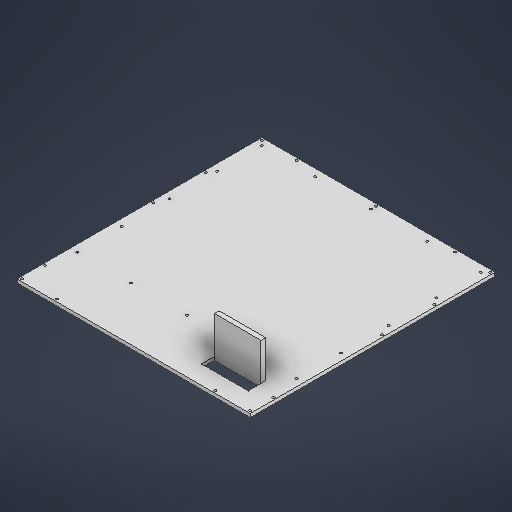
# Autodesk Inventor part: DesignAtasRobot
Saved by Autodesk Inventor 2026.1 (Build 301233020, 233B)
## iProperties
Created: 2025-11-08
Part Number: DesignAtasRobot
Material: Generic
Document SubType Name: Modeling
Designer: FrianVex
Density: 1 g/cm^3
Appearance: Default
Author: FrianVex
Autodesk Inventor part; units mm, degrees
ref_plane "YZ Plane" through (0, 0, 0) normal (1, 0, 0) x (0, 1, 0)
ref_plane "XZ Plane" through (0, 0, 0) normal (0, 1, 0) x (-1, 0, 0)
ref_plane "XY Plane" through (0, 0, 0) normal (0, 0, 1) x (1, 0, 0)
sketch "Sketch1" plane through (0, 0, 0) normal (0, 1, 0) x (-1, 0, 0)
  line L0 (100, -105) -> (-100, -105)
  line L1 (-100, -105) -> (-100, 105)
  line L2 (-100, 105) -> (100, 105)
  line L3 (100, 105) -> (100, -105)
  line L4 (100, -105) -> (-100, 105) construction
  line L5 (-100, -105) -> (100, 105) construction
  line L6 (-42.3092, 89.0348) -> (-82.3092, 89.0348)
  line L7 (-82.3092, 89.0348) -> (-82.3092, 74.0348)
  line L8 (-82.3092, 74.0348) -> (-42.3092, 74.0348)
  line L9 (-42.3092, 74.0348) -> (-42.3092, 89.0348)
  line L10 (-42.3092, 89.0348) -> (-82.3092, 74.0348) construction
  line L11 (-82.3092, 89.0348) -> (-42.3092, 74.0348) construction
  circle A0 centre (98, 83) radius 1
  circle A1 centre (98, 102.9) radius 1
  circle A2 centre (68, 102.9) radius 1
  circle A3 centre (-98, 102.9) radius 1
  circle A4 centre (-68, 102.9) radius 1
  circle A5 centre (98, -10) radius 1
  circle A6 centre (98, -55) radius 1
  circle A7 centre (-98, 83) radius 1
  circle A8 centre (-98, -10) radius 1
  circle A9 centre (-98, -55) radius 1
  circle A10 centre (-98, -102.9) radius 1.0002
  circle A11 centre (98, -102.9) radius 1
  circle A12 centre (-68, -102.9) radius 1
  circle A13 centre (0, -102.9) radius 1
  circle A14 centre (68, -102.9) radius 1
  line L12 (96, 61.2) -> (96, -100.8)
  circle A15 centre (94, -98.8) radius 1
  circle A16 centre (-94, -98.8) radius 1
  circle A17 centre (-94, 59.2) radius 1
  circle A18 centre (94, 59.2) radius 1
  circle A19 centre (94, -60.8) radius 1
  circle A20 centre (94, -19.8) radius 1
  circle A21 centre (94, 21.2) radius 1
  circle A22 centre (-94, -60.8) radius 1
  circle A23 centre (-94, -19.8) radius 1
  circle A24 centre (-94, 21.2) radius 1
  circle A25 centre (0, 59.2) radius 1
  circle A26 centre (0, -98.8) radius 1
  circle A27 centre (-48, 59.2) radius 1
  circle A28 centre (-48, -98.8) radius 1
  circle A29 centre (48, 59.2) radius 1
  circle A30 centre (48, -98.8) radius 1
  point P0 (0, 0)
  point P1 (-62.3092, 81.5348)
  dimension "d0" = 200
  dimension "d1" = 210
  dimension "d2" = 40
  dimension "d3" = 15
  dimension "d6" = 2
  dimension "d7" = 22
  dimension "d8" = 2
  dimension "d9" = 2
  dimension "d10" = 2.1
  dimension "d11" = 2
  dimension "d12" = 32
  dimension "d13" = 2.1
  dimension "d14" = 2
  dimension "d15" = 2.1
  dimension "d16" = 2
  dimension "d17" = 32
  dimension "d18" = 2.1
  dimension "d19" = 2
  dimension "d20" = 2
  dimension "d21" = 95
  dimension "d22" = 2
  dimension "d23" = 50
  dimension "d24" = 2
  dimension "d25" = 22
  dimension "d26" = 2
  dimension "d27" = 2
  dimension "d28" = 2
  dimension "d29" = 95
  dimension "d30" = 2
  dimension "d31" = 2
  dimension "d32" = 50
  dimension "d33" = 2
  dimension "d34" = 2.1
  dimension "d35" = 2.0005
  dimension "d36" = 2
  dimension "d38" = 2.1
  dimension "d39" = 2
  dimension "d40" = 32
  dimension "d41" = 2.1
  dimension "d42" = 2
  dimension "d43" = 2.1
  dimension "d44" = 100
  dimension "d45" = 2
  dimension "d46" = 2.1
  dimension "d47" = 32
  dimension "d56" = 2
  dimension "d59" = 6
  dimension "d60" = 6.2
  dimension "d61" = 2
  dimension "d64" = 6.2
  dimension "d65" = 6
  dimension "d66" = 2
  dimension "d69" = 6
  dimension "d70" = 45.8
  dimension "d71" = 2
  dimension "d74" = 6
  dimension "d75" = 45.8
  dimension "d77" = 2
  dimension "d79" = 2
  dimension "d80" = 2
  dimension "d84" = 2
  dimension "d87" = 2
  dimension "d90" = 2
  dimension "d93" = 2
  constraints: 31 centre point, 26 end point, 4 midpoint, 4 parallel, 4 point on line, 2 horizontal, 2 perpendicular
  measures "d0" distance of L1.end L2.end
  measures "d1" distance of L2.end L0.start
  measures "d2" distance of L8.end L7.end
  measures "d3" distance of L6.end L7.end
  measures "d6" diameter of A0
  measures "d7" distance from line of L2 A0.centre
  measures "d8" distance from line of L3 A0.centre
  measures "d9" diameter of A1
  measures "d10" distance from line of L2 A1.centre
  measures "d11" diameter of A2
  measures "d12" distance from line of L3 A2.centre
  measures "d13" distance from line of L2 A2.centre
  measures "d14" diameter of A3
  measures "d15" distance from line of L2 A3.centre
  measures "d16" diameter of A4
  measures "d17" distance from line of L1 A4.centre
  measures "d18" distance from line of L2 A4.centre
  measures "d19" diameter of A5
  measures "d20" distance from line of L3 A5.centre
  measures "d21" distance from line of L0 A5.centre
  measures "d22" diameter of A6
  measures "d23" distance from line of L0 A6.centre
  measures "d24" distance from line of L3 A6.centre
  measures "d25" distance from line of L2 A7.centre
  measures "d26" distance from line of L1 A7.centre
  measures "d27" diameter of A7
  measures "d28" diameter of A8
  measures "d29" distance from line of L0 A8.centre
  measures "d30" distance from line of L1 A8.centre
  measures "d31" diameter of A9
  measures "d32" distance from line of L0 A9.centre
  measures "d33" distance from line of L1 A9.centre
  measures "d34" distance from line of L0 A10.centre
  measures "d35" diameter of A10
  measures "d36" diameter of A11
  measures "d38" distance from line of L0 A11.centre
  measures "d39" diameter of A12
  measures "d40" distance from line of L1 A12.centre
  measures "d41" distance from line of L0 A12.centre
  measures "d42" diameter of A13
  measures "d43" distance from line of L0 A13.centre
  measures "d44" distance from line of L1 A13.centre
  measures "d45" diameter of A14
  measures "d46" distance from line of L0 A14.centre
  measures "d47" distance from line of L3 A14.centre
  measures "d56" diameter of A15
  measures "d59" distance from line of L3 A15.centre
  measures "d60" distance from line of L0 A15.centre
  measures "d61" diameter of A16
  measures "d64" distance from line of L0 A16.centre
  measures "d65" distance from line of L1 A16.centre
  measures "d66" diameter of A17
  measures "d69" distance from line of L1 A17.centre
  measures "d70" distance from line of L2 A17.centre
  measures "d71" diameter of A18
  measures "d74" distance from line of L3 A18.centre
  measures "d75" distance from line of L2 A18.centre
  measures "d77" diameter of A19
  measures "d79" diameter of A20
  measures "d80" diameter of A21
  measures "d84" diameter of A22
  measures "d87" diameter of A23
  measures "d90" diameter of A24
  measures "d93" diameter of A25
extrude "MainBody" add sketch "Sketch1" along normal blind 3
sketch "Sketch2" plane through (0, 3, 0) normal (0, 1, 0) x (1, 0, 0)
  line L0 (82.3092, -74.0348) -> (82.3092, -89.0348) projected
  line L1 (82.3092, -74.0348) -> (42.3092, -74.0348)
  line L2 (42.3092, -74.0348) -> (42.3092, -78.0348)
  line L3 (42.3092, -78.0348) -> (82.3092, -78.0348)
  line L4 (82.3092, -78.0348) -> (82.3092, -74.0348)
  point P0 (0, 0)
  dimension "d48" = 4
  dimension "d49" = 40
  constraints: 8 end point, 2 parallel, 1 horizontal, 1 perpendicular
  measures "d48" distance of L1.end L2.end
  measures "d49" distance of L2.end L3.end
extrude "Extrusion2" add sketch "Sketch2" along normal blind 32 and the other way blind 3
body "Solid1"
